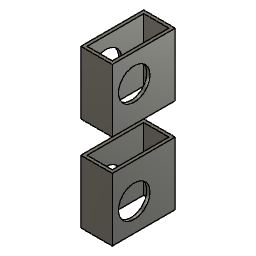
1x2+Aluminum+bar+with+hole+for+intake (Autodesk Fusion 360 design; units mm, degrees)
Autodesk Fusion 360 part; units mm, degrees
sketch "Sketch1" plane through (0, 0, 0) normal (0, 1, 0) x (1, 0, 0) in component "Component"
  line L0 (0, 0) -> (25.4, 0)
  line L1 (25.4, 0) -> (25.4, 50.8)
  line L2 (25.4, 50.8) -> (0, 50.8)
  line L3 (0, 50.8) -> (0, 0)
  line L4 (0, 50.8) -> (25.4, 0) construction
  line L5 (2.54, 2.54) -> (22.86, 2.54)
  line L6 (22.86, 2.54) -> (22.86, 48.26)
  line L7 (22.86, 48.26) -> (2.54, 48.26)
  line L8 (2.54, 48.26) -> (2.54, 2.54)
  line L9 (2.54, 2.54) -> (22.86, 48.26) construction
  line L10 (22.86, 2.54) -> (2.54, 48.26) construction
  point P0 (12.7, 25.4)
  dimension "d1" = 25.4
  dimension "d2" = 50.8
  dimension "d3" = 20.32
  dimension "d4" = 45.72
  constraint horizontal L0
  constraint vertical L1
  constraint horizontal L2
  constraint vertical L3
  constraint horizontal L5
  constraint perpendicular L5 L6
  constraint parallel L5 L7
  constraint parallel L6 L8
  constraint coincident L9 P0
  constraint coincident L10 P0
  constraint midpoint L4 P0
  measures "d1" distance of L0.start L0.end
  measures "d2" distance of L0.start L2.end
  measures "d3" distance of L6.end L7.end
  measures "d4" distance of L5.end L6.end
extrude "Extrude1" add sketch "Sketch1" along normal blind 50.8 makes body 1 in component "Component"
move_body "Move1" bodies 1 to x (1, 0, 0) y (0, 1, 0) z (0, 0, 1) at (0, 50.8, 0) in component "Component"
sketch "Sketch2" plane through (25.4, 0, 0) normal (1, 0, 0) x (0, 0, -1) in component "Component"
  line L0 (0, 50.8) -> (50.8, 50.8)
  line L1 (50.8, 50.8) -> (50.8, 101.6)
  line L2 (50.8, 101.6) -> (0, 101.6)
  line L3 (0, 101.6) -> (0, 50.8)
  circle A0 centre (17.7292, 73.3298) radius 12.7
  point P0 (17.7292, 73.3298)
  dimension "d7" = 22.5298
  dimension "d8" = 17.7292
  dimension "d9" = 25.4
  constraint coincident P0 A0.centre
  measures "d7" distance of L0 P0
  measures "d8" distance of L3 P0
  measures "d9" diameter of A0
extrude "Extrude2" cut sketch "Sketch2" against normal blind 6.35 contours A0 bodies 1 in component "Component"
sketch "Sketch3" plane through (0, 0, 0) normal (-1, 0, 0) x (0, 0, 1) in component "Component"
  line L0 (-50.8, 50.8) -> (0, 50.8)
  line L1 (0, 50.8) -> (0, 101.6)
  line L2 (0, 101.6) -> (-50.8, 101.6)
  line L3 (-50.8, 101.6) -> (-50.8, 50.8)
  circle A0 centre (-17.7292, 73.3298) radius 12.7
  point P0 (-17.7292, 73.3298)
  dimension "d12" = 22.5298
  dimension "d13" = 17.7292
  dimension "d14" = 25.4
  constraint coincident P0 A0.centre
  measures "d12" distance of L0 P0
  measures "d13" distance of L1 P0
  measures "d14" diameter of A0
extrude "Extrude3" cut sketch "Sketch3" against normal blind 6.35 contours A0 bodies 1 in component "Component"
mirror "Mirror1" about plane through (0, 101.6, 0) normal (0, 1, 0) of bodies 1 makes body 2 in component "Component"
move_body "Move2" bodies 2 to x (1, 0, 0) y (0, 1, 0) z (0, 0, 1) at (0, 25.4, 0) in component "Component"
component "Component" placed x (1, 0, 0) y (0, 1, 0) z (0, 0, 1) at (0, 0, 0)
